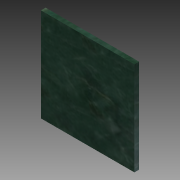
# Autodesk Inventor part: Base_01
Saved by Autodesk Inventor 2013 (Build 170138000, 138)
## iProperties
Created: 2008-06-06
Part Number: Base_01
Document SubType Name: Modeling
Designer: Phillip Dollan
Density: 1 g/cm^3
Material: Generic
Author: Phillip Dollan
Autodesk Inventor part; units mm, degrees
ref_plane "YZ Plane" through (0, 0, 0) normal (1, 0, 0) x (0, 1, 0)
ref_plane "XZ Plane" through (0, 0, 0) normal (0, 1, 0) x (-1, 0, 0)
ref_plane "XY Plane" through (0, 0, 0) normal (0, 0, 1) x (1, 0, 0)
sketch "Sketch1" plane through (0, 0, 0) normal (0, 0, 1) x (1, 0, 0)
  line L0 (51.4223, 276.9093) -> (-75.5777, 276.9093)
  line L1 (-75.5777, 276.9093) -> (-75.5777, 149.9093)
  line L2 (-75.5777, 149.9093) -> (51.4223, 149.9093)
  line L3 (51.4223, 149.9093) -> (51.4223, 276.9093)
  line L4 (-12.0777, -137.3102) -> (-12.0777, 23.761)
  line L5 (-12.0777, 23.761) -> (-12.0777, 149.9093) construction
  dimension "d0" = 127
  dimension "d1" = 127
  constraints: 12 end point, 2 parallel, 1 collinear, 1 horizontal, 1 midpoint, 1 perpendicular, 1 vertical, 2 other
  measures "d0" distance of L0.end L1.end
  measures "d1" distance of L0.start L0.end
extrude "Extrusion1" add sketch "Sketch1" against normal blind 6.35
ref_plane "Work Plane1" through (-75.5777, 213.4093, 0) normal (0, 1, 0) x (1, 0, 0)
ref_plane "Work Plane2" through (-12.0777, 149.9093, 0) normal (1, 0, 0) x (0, 0, -1)
body "Solid1"
